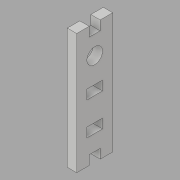
# Autodesk Inventor part: g_arm3
Saved by Autodesk Inventor 2019 (Build 230136000, 136)
## iProperties
Created: 2021-11-01
Part Number: g_arm3
Material: Generic
Document SubType Name: Modeling
Designer: Mohamed
Density: 1 g/cm^3
Appearance: Default
Author: Mohamed
Autodesk Inventor part; units mm, degrees
ref_plane "YZ Plane" through (0, 0, 0) normal (1, 0, 0) x (0, 1, 0)
ref_plane "XZ Plane" through (0, 0, 0) normal (0, 1, 0) x (-1, 0, 0)
ref_plane "XY Plane" through (0, 0, 0) normal (0, 0, 1) x (1, 0, 0)
sketch "Sketch1" plane through (0, 0, 0) normal (1, 0, 0) x (0, 1, 0)
  line L0 (0, 0) -> (77, 0)
  line L1 (77, 0) -> (77, -23)
  line L2 (77, -23) -> (0, -23)
  line L3 (0, -23) -> (0, 0)
  line L4 (71, -11.5) -> (71, -8)
  line L5 (71, -8) -> (71, -15)
  line L6 (71, -15) -> (77, -15)
  line L7 (71, -8) -> (77, -8)
  line L8 (0, -8) -> (6, -8)
  line L9 (6, -8) -> (6, -15)
  line L10 (6, -15) -> (0, -15)
  circle A0 centre (59, -11.5) radius 5
  dimension "d0" = 77
  dimension "d1" = 23
  dimension "d3" = 3.5
  dimension "d4" = 7
  dimension "d5" = 6
  dimension "d6" = 7
  dimension "d10" = 10
  constraints: 22 end point, 5 point on line, 4 perpendicular, 3 parallel, 2 horizontal, 1 centre point
  measures "d0" distance of L1.end L2.end
  measures "d1" distance of L0.end L1.end
  measures "d3" distance of L4.start L4.end
  measures "d4" distance of L4.end L5.end
  measures "d5" distance of L8.start L8.end
  measures "d6" distance of L8.end L9.end
  measures "d10" diameter of A0
extrude "Extrusion1" add sketch "Sketch1" along normal blind 6 contours L0 L1 L7 L4 L5 L6 L2 L3 L10 L9 L8 | A0
sketch "Sketch2" plane through (6, 0, 0) normal (1, 0, 0) x (0, 0, -1)
  line L0 (15, 71) -> (8, 71) projected
  circle A0 centre (11.5, 59) radius 5
  point P0 (0, 0)
  dimension "d12" = 10
  constraints: 1 centre point
  measures "d12" diameter of A0
extrude "Extrusion2" cut sketch "Sketch2" against normal blind 6
sketch "Sketch3" plane through (6, 0, 0) normal (1, 0, 0) x (0, 0, -1)
  line L0 (8, 6) -> (15, 6) projected
  line L1 (11.5, 16) -> (6.5, 16)
  line L2 (6.5, 16) -> (6.5, 22)
  line L3 (6.5, 22) -> (16.5, 22)
  line L4 (16.5, 22) -> (16.5, 16)
  line L5 (16.5, 16) -> (11.5, 16)
  line L6 (11.5, 37) -> (16.5, 37)
  line L7 (16.5, 37) -> (16.5, 43)
  line L8 (16.5, 43) -> (6.5, 43)
  line L9 (6.5, 43) -> (6.5, 37)
  line L10 (6.5, 37) -> (11.5, 37)
  point P0 (0, 0)
  dimension "d16" = 5
  dimension "d17" = 6
  dimension "d18" = 10
  dimension "d19" = 6
  dimension "d21" = 5
  dimension "d22" = 6
  dimension "d23" = 10
  dimension "d24" = 6
  constraints: 20 end point, 4 perpendicular, 2 horizontal, 2 point on line
  measures "d16" distance of L1.start L1.end
  measures "d17" distance of L1.end L2.end
  measures "d18" distance of L2.end L3.end
  measures "d19" distance of L3.end L4.end
  measures "d21" distance of L6.start L6.end
  measures "d22" distance of L6.end L7.end
  measures "d23" distance of L7.end L8.end
  measures "d24" distance of L8.end L9.end
extrude "Extrusion3" cut sketch "Sketch3" against normal blind 6
body "Solid1"
